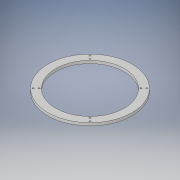
# Autodesk Inventor part: Slewing Bearing
Saved by Autodesk Inventor 2019.4 (Build 234330000, 330)
## iProperties
Created: 2020-01-06
Part Number: Slewing Bearing
Material: Generic
Document SubType Name: Modeling
Designer: admin
Density: 1 g/cm^3
Appearance: Default
Author: admin
Autodesk Inventor part; units mm, degrees
ref_plane "YZ Plane" through (0, 0, 0) normal (1, 0, 0) x (0, 1, 0)
ref_plane "XZ Plane" through (0, 0, 0) normal (0, 1, 0) x (-1, 0, 0)
ref_plane "XY Plane" through (0, 0, 0) normal (0, 0, 1) x (1, 0, 0)
sketch "Sketch1" plane through (0, 0, 0) normal (0, 1, 0) x (-1, 0, 0)
  circle A0 centre (0, 0) radius 122.5
  circle A1 centre (0, 0) radius 150
  line L0 (-91, 91) -> (91, 91) construction
  line L1 (91, 91) -> (91, -91) construction
  line L2 (91, -91) -> (-91, -91) construction
  line L3 (-91, -91) -> (-91, 91) construction
  line L4 (-91, 91) -> (91, -91) construction
  line L5 (91, 91) -> (-91, -91) construction
  line L6 (-101.5, 101.5) -> (101.5, 101.5) construction
  line L7 (101.5, 101.5) -> (101.5, -101.5) construction
  line L8 (101.5, -101.5) -> (-101.5, -101.5) construction
  line L9 (-101.5, -101.5) -> (-101.5, 101.5) construction
  line L10 (-101.5, 101.5) -> (101.5, -101.5) construction
  line L11 (101.5, 101.5) -> (-101.5, -101.5) construction
  circle A2 centre (-101.5, 101.5) radius 2.75
  circle A3 centre (-91, 91) radius 2.75
  circle A4 centre (-101.5, -101.5) radius 2.75
  circle A5 centre (-91, -91) radius 2.75
  circle A6 centre (91, -91) radius 2.75
  circle A7 centre (101.5, -101.5) radius 2.75
  circle A8 centre (91, 91) radius 2.75
  circle A9 centre (101.5, 101.5) radius 2.75
  dimension "d0" = 245
  dimension "d1" = 300
  dimension "d2" = 182
  dimension "d3" = 203
  dimension "d4" = 5.5
  dimension "d5" = 5.5
  dimension "d6" = 5.5
  dimension "d7" = 5.5
  dimension "d8" = 5.5
  dimension "d9" = 5.5
  dimension "d10" = 5.5
  dimension "d11" = 5.5
  constraints: 24 end point, 10 centre point, 10 coincident, 4 midpoint, 4 parallel, 3 perpendicular, 2 horizontal, 1 point on line
  measures "d0" diameter of A0
  measures "d1" diameter of A1
  measures "d2" distance of L2.end L0.start
  measures "d3" distance of L8.end L6.start
  measures "d4" diameter of A2
  measures "d5" diameter of A3
  measures "d6" diameter of A4
  measures "d7" diameter of A5
  measures "d8" diameter of A6
  measures "d9" diameter of A7
  measures "d10" diameter of A8
  measures "d11" diameter of A9
extrude "Extrusion1" add sketch "Sketch1" along normal blind 10
body "Solid1"
